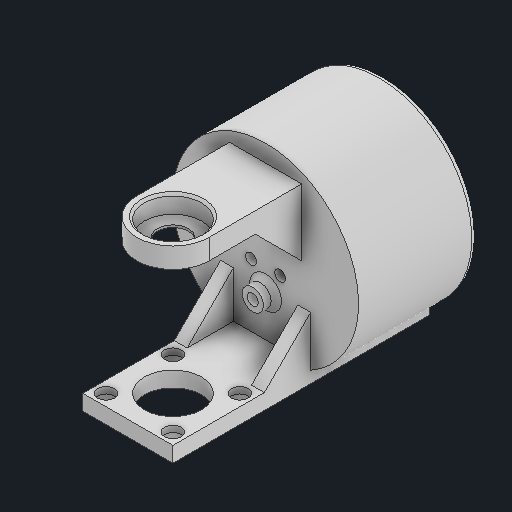
# Autodesk Inventor part: j4 moving part
Saved by Autodesk Inventor 2026.1 (Build 301233020, 233B)
## iProperties
Created: 2025-08-05
Part Number: j4 moving part
Material: 一般
Document SubType Name: Modeling
Designer: gavin
Density: 1 g/cm^3
Appearance: 預設
Author: gavin
## iProperties of the stored document j4 moving part_3D 列印.ipt
Created: 2025-08-05
Part Number: j4 moving part_3D 列印
Material: 一般
Document SubType Name: Modeling
Designer: gavin
Density: 1 g/cm^3
Appearance: 預設
Author: gavin
Autodesk Inventor part; units mm, degrees
sketch "草圖1" plane through (0, 0, 0) normal (0, 0, 1) x (1, 0, 0)
  circle A0 centre (0, 0) radius 31.075
  circle A1 centre (0, 0) radius 36.075
  dimension "d0" = 62.15
  dimension "d1" = 5
  constraints: 2 centre point, 1 coincident
  measures "d0" diameter of A0
  measures "d1" radial gap between concentric circles of A0 A1
ref_plane "工作平面1" through (-29.6675, -29.6675, -41) normal (0, 0, -1) x (-0.0056937, 0.9999838, 0)
extrude "擠出1" add sketch "草圖1" against normal up to surface (41 mm away)
sketch "草圖2" plane through (0, 0, 0) normal (0, 0, 1) x (1, 0, 0)
  circle A0 centre (0, 0) radius 36.075 projected
  circle A1 centre (0, 0) radius 31.075 projected
  circle A2 centre (0, 0) radius 28.075
  dimension "d4" = 3
  constraints: 1 centre point
  measures "d4" radial gap between concentric circles of A1 A2
ref_plane "工作平面2" through (-29.6675, -29.6675, -27) normal (0, 0, 1) x (0.9999838, 0.0056937, 0)
extrude "擠出2" add sketch "草圖2" against normal up to surface (27 mm away) contours A1
sketch "草圖3" plane through (0, 0, 0) normal (0, 0, 1) x (1, 0, 0)
  circle A0 centre (0, 0) radius 28.075 projected
  circle A1 centre (0, 0) radius 36.075 projected
extrude "擠出3" add sketch "草圖3" along normal blind 5 contours A0 | A1
sketch "草圖4" plane through (0, 0, 5) normal (0, 0, 1) x (1, 0, 0)
  circle A0 centre (0, 0) radius 8 construction
  line L0 (0, 0) -> (-5.6569, 5.6569) construction
  line L1 (0, 0) -> (8, 0) construction
  circle A1 centre (-5.6569, 5.6569) radius 2.1
  circle A2 centre (-5.6569, -5.6569) radius 2.1
  circle A3 centre (5.6569, -5.6569) radius 2.1
  circle A4 centre (5.6569, 5.6569) radius 2.1
  dimension "d9" = 16
  dimension "d17" = 135
  dimension "d18" = 4.2
  dimension "d21" = 360
  constraints: 5 coincident, 4 centre point, 4 end point, 1 equal length, 1 horizontal, 16 other
  measures "d17" angle of L1 L0
  measures "d18" diameter of A1
extrude "擠出4" cut sketch "草圖4" against normal blind 5
sketch "草圖5" plane through (0, 0, 5) normal (0, 0, 1) x (1, 0, 0)
  circle A0 centre (0, -14) radius 2.165
  circle A1 centre (0, 14) radius 2.165
  circle A2 centre (0, -14) radius 4.165
  circle A3 centre (0, 14) radius 4.165
  point P0 (0, 0)
  dimension "d23" = 4.33
  dimension "d24" = 4.33
  dimension "d25" = 14
  dimension "d26" = 28
  dimension "d27" = 2
  dimension "d28" = 2
  constraints: 4 centre point
  measures "d23" diameter of A0
  measures "d24" diameter of A1
  measures "d25" distance of point (0, 0) A1.centre
  measures "d26" distance of A0.centre A1.centre
  measures "d27" radial gap between concentric circles of A0 A2
  measures "d28" radial gap between concentric circles of A1 A3
extrude "擠出5" add sketch "草圖5" along normal blind 5
sketch "草圖6" plane through (0, -14, 10) normal (0, 0, 1) x (1, 0, 0)
  circle A0 centre (0, 0) radius 2.165 projected
  circle A1 centre (0, 28) radius 2.165 projected
  point P0 (0, 14)
extrude "擠出6" cut sketch "草圖6" against normal through all
fillet "圓角1" radius 2 2 edges at (-4.165, -14, 5) (-4.165, 14, 5)
sketch "草圖7" plane through (0, 0, 5) normal (0, 0, 1) x (1, 0, 0)
  line L0 (17.5, -36.075) -> (-17.5, -36.075)
  line L1 (-17.5, -36.075) -> (-17.5, -30.075)
  line L2 (-17.5, -30.075) -> (17.5, -30.075)
  line L3 (17.5, -30.075) -> (17.5, -36.075)
  line L4 (17.5, -36.075) -> (-17.5, -30.075) construction
  line L5 (-17.5, -36.075) -> (17.5, -30.075) construction
  line L6 (0, 0) -> (0, -36.075) construction
  circle A0 centre (0, 0) radius 36.075 construction
  circle A1 centre (0, 0) radius 36.075 projected
  point P0 (0, -33.075)
  dimension "d34" = 35
  dimension "d35" = 6
  dimension "d37" = 36.075
  constraints: 14 end point, 2 horizontal, 2 midpoint, 2 parallel, 2 vertical alignment, 1 perpendicular, 1 point on line, 1 vertical, 1 other
  measures "d34" distance of L0.start L0.end
  measures "d35" distance of L0.end L1.end
  measures "d37" distance from line of L6.start L0
extrude "擠出7" add sketch "草圖7" along normal blind 53.5 contours L0 A1 L3 | L0 L1 A1 | A1 L1 L2 L3 picked at (-2.0205, -31.904)
sketch "草圖8" plane through (-17.5, -36.075, 5) normal (0, -1, 0) x (1, 0, 0)
  line L0 (35, 0) -> (35, 53.5) projected
  line L1 (0, 53.5) -> (35, 53.5) projected
  line L2 (0, 0) -> (0, 53.5) projected
  line L3 (30.5, 23) -> (4.5, 23) construction
  line L4 (4.5, 23) -> (4.5, 49) construction
  line L5 (4.5, 49) -> (30.5, 49) construction
  line L6 (30.5, 49) -> (30.5, 23) construction
  line L7 (30.5, 23) -> (4.5, 49) construction
  line L8 (4.5, 23) -> (30.5, 49) construction
  circle A0 centre (4.5, 23) radius 1.6
  circle A1 centre (30.5, 23) radius 1.6
  circle A2 centre (30.5, 49) radius 1.6
  circle A3 centre (4.5, 49) radius 1.6
  circle A4 centre (17.5, 36) radius 11.075
  line L9 (0, 0) -> (17.5, 0) projected
  line L10 (17.5, 0) -> (35, 0) projected
  point P0 (17.5, -5)
  dimension "d40" = 26
  dimension "d41" = 26
  dimension "d42" = 4.5
  dimension "d43" = 4.5
  dimension "d44" = 3.2
  dimension "d47" = 360
  dimension "d57" = 22.15
  constraints: 12 end point, 5 centre point, 2 coincident, 2 midpoint, 2 parallel, 1 horizontal, 1 perpendicular, 9 other
  measures "d40" distance of L4.end L5.end
  measures "d41" distance of L3.end L4.end
  measures "d42" distance between parallel lines of L1 L5
  measures "d43" distance between parallel lines of L0 L6
  measures "d44" diameter of A0
  measures "d57" diameter of A4
extrude "擠出8" cut sketch "草圖8" against normal up to surface (6 mm away) contours A0 | A1 | A2 | A3 | A4
sketch "草圖9" plane through (-17.5, -30.075, 5) normal (0, 1, 0) x (1, 0, 0)
  circle A0 centre (30.5, -23) radius 1.6 projected
  circle A1 centre (4.5, -23) radius 1.6 projected
  circle A2 centre (30.5, -49) radius 1.6 projected
  circle A3 centre (4.5, -49) radius 1.6 projected
  line L0 (0, 0) -> (35, 0) projected
  line L1 (0, 0) -> (0, -53.5) projected
  line L2 (35, -53.5) -> (0, -53.5) projected
  line L3 (35, 0) -> (35, -53.5) projected
  circle A4 centre (4.5, -23) radius 3.25
  circle A5 centre (30.5, -23) radius 3.25
  circle A6 centre (30.5, -49) radius 3.25
  circle A7 centre (4.5, -49) radius 3.25
  point P0 (17.5, 5)
  dimension "d51" = 6.5
  dimension "d52" = 6.5
  dimension "d53" = 6.5
  dimension "d54" = 6.5
  constraints: 4 centre point, 4 coincident
  measures "d51" diameter of A4
  measures "d52" diameter of A5
  measures "d53" diameter of A6
  measures "d54" diameter of A7
extrude "擠出9" cut sketch "草圖9" against normal blind 2.5 contours A3 | A4 | A5 | A6 | A7
sketch "草圖10" plane through (0, 0, 5) normal (0, 0, 1) x (1, 0, 0)
  line L0 (-14, 21.475) -> (14, 21.475)
  line L1 (14, 21.475) -> (14, 29.375)
  line L2 (14, 29.375) -> (-14, 29.375)
  line L3 (-14, 29.375) -> (-14, 21.475)
  line L4 (-14, 21.475) -> (14, 29.375) construction
  line L5 (14, 21.475) -> (-14, 29.375) construction
  line L6 (-10.6499, -2.75) -> (-13.9992, -2.75) projected
  line L7 (-13.9992, -2.75) -> (-13.9992, -18) projected
  line L8 (-13.9992, -18) -> (14.0008, -18) projected
  line L9 (14.0008, -18) -> (14.0008, 20.075) projected
  line L10 (-13.9992, 20.075) -> (14.0008, 20.075) projected
  line L11 (-13.9992, 2.75) -> (-13.9992, 20.075) projected
  line L12 (-13.9992, 2.75) -> (-10.6499, 2.75) projected
  ellipse E0 centre (0.0008, 0) end of major axis (0.0008, -11) minor radius 11 (-10.6499, -2.75) -> (-10.6499, 2.75) ccw projected
  ellipse E1 centre (-11.4992, 11.5) end of major axis (-11.4992, 10.15) minor radius 1.35 projected
  ellipse E2 centre (11.5008, 11.5) end of major axis (11.5008, 10.15) minor radius 1.35 projected
  ellipse E3 centre (11.5008, -11.5) end of major axis (11.5008, -12.85) minor radius 1.35 projected
  ellipse E4 centre (-11.4992, -11.5) end of major axis (-11.4992, -12.85) minor radius 1.35 projected
  point P0 (0, 0)
  point P1 (0, 25.425)
  dimension "d59" = 28
  dimension "d60" = 7.9
  dimension "d61" = 1.4
  constraints: 12 end point, 2 midpoint, 2 parallel, 1 horizontal, 1 perpendicular, 1 other
  measures "d59" distance of L2.end L1.end
  measures "d60" distance of L1.end L0.end
  measures "d61" distance between parallel lines of L10 L0
extrude "擠出10" add sketch "草圖10" along normal blind 50 contours L3 L2 L1 L0
sketch "草圖11" plane through (-14, 29.375, 5) normal (0, 1, 0) x (1, 0, 0)
  circle A0 centre (14, -36) radius 11.075 projected
  circle A1 centre (14, -36) radius 11.075
  point P0 (14, 5)
  point P1 (19.9074, -23.1321)
  point P2 (19.5786, -46.8782)
  point P3 (23.3679, -26.5926)
  dimension "d64" = 22.15
  constraints: 1 coincident, 3 other
extrude "擠出11" cut sketch "草圖11" against normal blind 7
sketch "草圖12" plane through (0, 22.375, 41) normal (0, 1, 0) x (1, 0, 0)
  circle A0 centre (0, 0) radius 6
  point P0 (0, 41)
  dimension "d67" = 12
  constraints: 1 centre point
  measures "d67" diameter of A0
extrude "擠出12" cut sketch "草圖12" against normal up to surface (0.9 mm away)
chamfer "倒角1" distance 0.9 angle 45 1 edges at (-11.075, 29.375, 41)
ref_plane "工作平面3" through (0, -36.075, 0) normal (0, 1, 0) x (-1, 0, 0)
chamfer "倒角2" distance 1.65 angle 45 4 edges at (-14.6, -32.575, 28) (11.4, -32.575, 28) (11.4, -32.575, 54) (-14.6, -32.575, 54)
sketch "草圖19" plane through (0, 0, 5) normal (0, 0, -1) x (-1, 0, 0)
  line L0 (-14.4818, -38.575) -> (-11.4818, -38.575) projected
  arc A0 (-17.5, -31.5461) -> (0, -36.075) centre (0, 0) ccw projected
  line L1 (-17.5, -36.075) -> (-17.5, -31.5461) projected
  line L2 (0, -36.075) -> (-17.5, -36.075) projected
  arc A1 (0, -36.075) -> (17.5, -31.5461) centre (0, 0) ccw projected
  line L3 (17.5, -36.075) -> (0, -36.075) projected
  line L4 (17.5, -31.5461) -> (17.5, -36.075) projected
  point P0 (0, -36.075)
  point P1 (0, -36.075)
  point P2 (0, -36.075)
  point P3 (0, -36.075)
extrude "擠出19" add sketch "草圖19" along normal up to surface (46 mm away)
sketch "草圖20" plane through (-17.5, -36.075, -41) normal (0, -1, 0) x (1, 0, 0)
  circle A0 centre (4.5, 95) radius 1.6 projected
  circle A1 centre (17.5, 82) radius 11.075 projected
  circle A2 centre (30.5, 95) radius 1.6 projected
  circle A3 centre (4.5, 69) radius 1.6 projected
  circle A4 centre (30.5, 69) radius 1.6 projected
  line L0 (0, 0) -> (0, 99.5) projected
  line L1 (0, 0) -> (35, 0) projected
  line L2 (35, 0) -> (35, 99.5) projected
  line L3 (0, 99.5) -> (35, 99.5) projected
  circle A5 centre (17.5, 5) radius 2.165
  point P0 (17.5, 41)
  dimension "d103" = 4.33
  dimension "d104" = 5
  constraints: 1 centre point
  measures "d103" diameter of A5
  measures "d104" distance from line of L1 A5.centre
extrude "擠出20" cut sketch "草圖20" against normal blind 10 contours A5
sketch "草圖21" plane through (-14, 21.475, 5) normal (-1, 0, 0) x (0, 0, 1)
  line L0 (0, 0) -> (50, 0) projected
  line L1 (0, -53.0211) -> (0, 14.6) projected
  line L2 (18, 0) -> (0, -18)
  point P0 (-5, -21.475)
  point P1 (53.5, 0)
  point P2 (0, -57.55)
  dimension "d107" = 45
  dimension "d108" = 18
  constraints: 2 end point, 2 point on line
  measures "d107" angle of L0 L2
  measures "d108" distance from line of L1 L2.start
extrude "擠出21" add sketch "草圖21" against normal blind 5
mirror "鏡射2" about plane through (0, 0, 0) normal (1, 0, 0) of "擠出21"
sketch "草圖22" plane through (-17.5, -36.075, 58.5) normal (-1, 0, 0) x (0, 0, 1)
  line L0 (-53.5, 4.5289) -> (-53.5, 6) projected
  line L1 (-99.5, 4.5289) -> (-53.5, 4.5289) projected
  line L2 (-99.5, 4.5289) -> (-99.5, 0) projected
  line L3 (-99.5, 0) -> (0, 0) projected
  line L4 (0, 6) -> (0, 0) projected
  line L5 (-53.5, 6) -> (0, 6) projected
  line L6 (-53.5, 4.5289) -> (-53.5, 72.15) projected
  line L7 (-35.5, 6) -> (-53.5, 24)
  point P0 (-58.5, 36.075)
  dimension "d111" = 45
  dimension "d112" = 18
  constraints: 2 end point, 2 point on line
  measures "d111" angle of L5 L7
  measures "d112" distance from line of L6 L7.start
extrude "擠出22" add sketch "草圖22" against normal blind 5 contours L6 L7 L5
mirror "鏡射3" about plane through (0, 0, 0) normal (1, 0, 0) of "擠出22"
fillet "圓角5" radius 2 1 edges at (0, 36.075, -41)
fillet "圓角6" radius 14 2 edges at (-14, 25.425, 55) (14, 25.425, 55)
equation "\"d40\" = d41"
equation "\"d52\" = d51"
equation "\"d53\" = d52"
equation "\"d54\" = d51"
